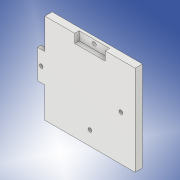
# Autodesk Inventor part: TC001
Saved by Autodesk Inventor 2017 SP1 (Build 210196100, 196)
## iProperties
Created: 2017-08-15
Part Number: TC001
Material: ABS Plastic
Document SubType Name: Modeling
Designer: Zach
Density: 1.06 g/cm^3
Appearance: CR White
Author: Zach
Autodesk Inventor part; units mm, degrees
ref_plane "YZ Plane" through (0, 0, 0) normal (1, 0, 0) x (0, 1, 0)
ref_plane "XZ Plane" through (0, 0, 0) normal (0, 1, 0) x (-1, 0, 0)
ref_plane "XY Plane" through (0, 0, 0) normal (0, 0, 1) x (1, 0, 0)
sketch "Sketch1" plane through (0, 0, 0) normal (0, 0, 1) x (1, 0, 0)
  line L0 (0, 0) -> (124, 0)
  line L1 (124, 0) -> (124, 124)
  line L2 (124, 124) -> (0, 124)
  line L3 (0, 124) -> (0, 0)
  dimension "d0" = 124
  dimension "d1" = 124
  constraints: 8 end point, 2 parallel, 1 horizontal, 1 perpendicular
  measures "d0" distance of L2.end L1.end
  measures "d1" distance of L1.end L0.end
extrude "Extrusion1" add sketch "Sketch1" along normal blind 10
sketch "Sketch2" plane through (0, 0, 10) normal (0, 0, 1) x (1, 0, 0)
  line L0 (124, 124) -> (0, 124) projected
  line L1 (41, 124) -> (83, 124)
  line L2 (83, 124) -> (83, 112)
  line L3 (83, 112) -> (41, 112)
  line L4 (41, 112) -> (41, 124)
  point P0 (0, 0)
  point P1 (62, 112)
  point P2 (62, 124)
  dimension "d4" = 42
  dimension "d5" = 12
  constraints: 8 end point, 2 midpoint, 2 parallel, 1 horizontal, 1 perpendicular, 1 point on line, 1 vertical alignment
  measures "d4" distance of L2.end L3.end
  measures "d5" distance of L1.end L2.end
extrude "Extrusion2" cut sketch "Sketch2" against normal blind 6
sketch "Sketch3" plane through (0, 0, 4) normal (0, 0, 1) x (1, 0, 0)
  circle A0 centre (62, 119) radius 2.5
  line L0 (41, 124) -> (83, 124) construction
  line L1 (41, 112) -> (41, 124) construction
  line L2 (83, 112) -> (41, 112) construction
  line L3 (83, 124) -> (83, 112) construction
  point P0 (0, 0)
  point P1 (62, 124)
  point P2 (83, 118)
  dimension "d8" = 5
  dimension "d22" = 5
  constraints: 2 midpoint, 1 centre point, 1 vertical alignment
  measures "d8" diameter of A0
  measures "d22" distance of A0.centre point (62, 124)
extrude "Extrusion3" cut sketch "Sketch3" against normal through all
sketch "Sketch4" plane through (0, 0, 10) normal (0, 0, 1) x (1, 0, 0)
  line L0 (0, 124) -> (0, 0) projected
  line L1 (0, 82) -> (-10, 82)
  line L2 (-10, 82) -> (-10, 42)
  line L3 (-10, 42) -> (0, 42)
  line L4 (0, 42) -> (0, 82)
  circle A0 centre (-5, 62) radius 2.5
  point P0 (-10, 62)
  point P1 (0, 62)
  point P2 (-5, 82)
  dimension "d11" = 10
  dimension "d12" = 40
  dimension "d13" = 5
  constraints: 8 end point, 3 midpoint, 2 horizontal alignment, 2 parallel, 1 centre point, 1 horizontal, 1 perpendicular, 1 point on line, 1 vertical alignment
  measures "d11" distance of L3.end L2.end
  measures "d12" distance of L2.end L1.end
  measures "d13" diameter of A0
extrude "Extrusion4" add sketch "Sketch4" against normal blind 5
sketch "Sketch5" plane through (0, 0, 10) normal (0, 0, 1) x (1, 0, 0)
  circle A0 centre (62, 19.5) radius 2.5
  line L0 (0, 0) -> (124, 0) projected
  circle A1 centre (104.5, 62) radius 2.5
  line L1 (124, 0) -> (124, 124) projected
  point P0 (62, 0)
  point P1 (124, 62)
  dimension "d16" = 5
  dimension "d17" = 19.5
  dimension "d18" = 5
  dimension "d19" = 19.5
  constraints: 2 centre point, 2 midpoint, 1 horizontal alignment, 1 vertical alignment
  measures "d16" diameter of A0
  measures "d17" distance from line of L0 A0.centre
  measures "d18" diameter of A1
  measures "d19" distance from line of L1 A1.centre
extrude "Extrusion5" cut sketch "Sketch5" against normal through all
body "Solid1"
